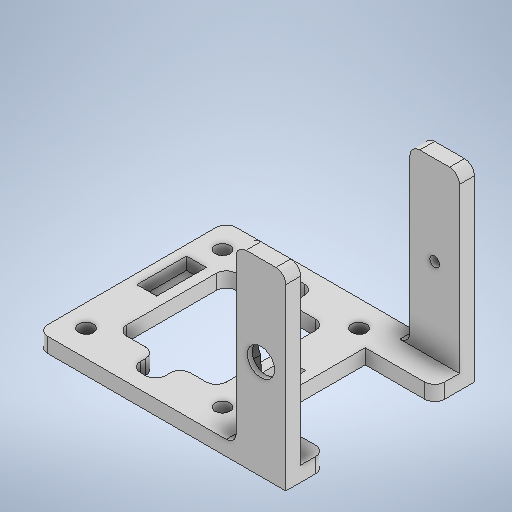
# Autodesk Inventor part: head_top
Saved by Autodesk Inventor 2026.1 (Build 301233000, 233)
## iProperties
Created: 2026-01-12
Part Number: head_top
Material: Generic
Document SubType Name: Modeling
Designer: chris
Density: 1 g/cm^3
Appearance: Default
Author: chris
Autodesk Inventor part; units mm, degrees
ref_plane "YZ Plane" through (0, 0, 0) normal (1, 0, 0) x (0, 1, 0)
ref_plane "XZ Plane" through (0, 0, 0) normal (0, 1, 0) x (-1, 0, 0)
ref_plane "XY Plane" through (0, 0, 0) normal (0, 0, 1) x (1, 0, 0)
sketch "Sketch1" plane through (0, 0, 0) normal (0, 1, 0) x (-1, 0, 0)
  line L0 (-25, 19) -> (25, 19)
  line L1 (25, 19) -> (25, -19)
  line L2 (25, -19) -> (-25, -19)
  line L3 (-25, -19) -> (-25, 19)
  line L4 (-25, 19) -> (25, -19) construction
  line L5 (25, 19) -> (-25, -19) construction
  line L6 (-15, -11) -> (25, -11)
  line L7 (25, -11) -> (25, 11)
  line L8 (25, 11) -> (-15, 11)
  line L9 (-15, 11) -> (-15, -11)
  line L10 (-15, -11) -> (25, 11) construction
  line L11 (25, -11) -> (-15, 11) construction
  point P0 (0, 0)
  point P1 (5, 0)
  point P2 (5, 0)
  point P3 (25, -11)
  point P4 (25, 11)
  dimension "d0" = 50
  dimension "d1" = 38
  dimension "d2" = 22
  dimension "d3" = 5
  dimension "d4" = 40
  constraints: 24 end point, 5 midpoint, 5 parallel, 2 perpendicular, 1 horizontal
  measures "d0" distance of L1.end L2.end
  measures "d1" distance of L0.end L1.end
  measures "d2" distance of L7.end L6.end
  measures "d3" distance of point (0, 0) point (5, 0)
  measures "d4" distance of L6.start L6.end
extrude "Extrusion1" add sketch "Sketch1" along normal blind 3 contours L0 L1 L8 L9 L6 L2 L3
sketch "Sketch2" plane through (0, 3, 0) normal (0, 1, 0) x (1, 0, 0)
  line L0 (25, -19) -> (15, -19)
  line L1 (15, -19) -> (15, -16)
  line L2 (15, -16) -> (25, -16)
  line L3 (25, -16) -> (25, -19)
  line L4 (-25, -19) -> (25, -19) projected
  line L5 (15, 11) -> (15, -11) projected
  line L6 (25, -19) -> (25, 19) projected
  line L7 (15, -11) -> (-25, -11) projected
  line L8 (15, 16) -> (25, 16)
  line L9 (25, 16) -> (25, 19)
  line L10 (25, 19) -> (15, 19)
  line L11 (15, 19) -> (15, 16)
  line L12 (-25, 11) -> (15, 11) projected
  line L13 (25, 19) -> (-25, 19) projected
  point P0 (0, 0)
  point P1 (25, 16)
  dimension "d18" = 3
  dimension "d19" = 3
  constraints: 16 end point, 6 collinear, 4 parallel, 2 horizontal, 2 perpendicular
  measures "d18" distance of L10.end L8.start
  measures "d19" distance of L0.end L1.end
extrude "Extrusion2" add sketch "Sketch2" along normal blind 35
sketch "Sketch4" plane through (25, 0, -19) normal (0, 0, -1) x (-1, 0, 0)
  circle A0 centre (5, 20) radius 1
  line L0 (0, 0) -> (50, 0) projected
  line L1 (0, 0) -> (0, 38) projected
  point P0 (25, 0)
  dimension "d20" = 2
  dimension "d21" = 20
  dimension "d22" = 5
  constraints: 1 centre point
  measures "d20" diameter of A0
  measures "d21" distance from line of A0.centre L0
  measures "d22" distance from line of L1 A0.centre
extrude "Extrusion4" cut sketch "Sketch4" against normal blind 5
sketch "Sketch6" plane through (0, 0, 0) normal (0, -1, 0) x (1, 0, 0)
  circle A0 centre (-20.5, 13.75) radius 1.5
  circle A1 centre (-20.5, -13.75) radius 1.5
  circle A2 centre (7, -13.75) radius 1.5
  circle A3 centre (7, 13.75) radius 1.5
  line L0 (-9.25, 16) -> (-4.25, 16)
  line L1 (-4.25, 16) -> (-4.25, 11)
  line L2 (-4.25, 11) -> (-9.25, 11)
  line L3 (-9.25, 11) -> (-9.25, 16)
  line L4 (-9.25, 16) -> (-4.25, 11) construction
  line L5 (-4.25, 16) -> (-9.25, 11) construction
  line L6 (15, 11) -> (-25, 11) projected
  line L7 (25, 19) -> (25, -19) projected
  line L8 (-9.25, -16) -> (-4.25, -16)
  line L9 (-4.25, -16) -> (-4.25, -11)
  line L10 (-4.25, -11) -> (-9.25, -11)
  line L11 (-9.25, -11) -> (-9.25, -16)
  line L12 (-9.25, -16) -> (-4.25, -11) construction
  line L13 (-4.25, -16) -> (-9.25, -11) construction
  line L14 (-25, -11) -> (15, -11) projected
  point P0 (0, 0)
  point P1 (-6.75, 13.5)
  point P2 (-6.75, -13.5)
  dimension "d43" = 3
  dimension "d44" = 3
  dimension "d45" = 3
  dimension "d46" = 3
  dimension "d47" = 13.75
  dimension "d48" = 13.75
  dimension "d49" = 13.75
  dimension "d50" = 13.75
  dimension "d51" = 27.5
  dimension "d52" = 27.5
  dimension "d55" = 5
  dimension "d56" = 5
  dimension "d57" = 13.75
  dimension "d58" = 18
  dimension "d59" = 18
  dimension "d60" = 5
  dimension "d61" = 5
  dimension "d62" = 13.75
  constraints: 24 end point, 4 centre point, 4 midpoint, 4 parallel, 2 collinear, 2 horizontal, 2 perpendicular
  measures "d43" diameter of A0
  measures "d44" diameter of A1
  measures "d45" diameter of A2
  measures "d46" diameter of A3
  measures "d47" vertical distance of A0.centre point (0, 0)
  measures "d48" vertical distance of point (0, 0) A1.centre
  measures "d49" vertical distance of A2.centre point (0, 0)
  measures "d50" vertical distance of A3.centre point (0, 0)
  measures "d51" distance of A2.centre A1.centre
  measures "d52" distance of A3.centre A0.centre
  measures "d55" distance of L0.end L1.end
  measures "d56" distance of L0.start L0.end
  measures "d57" horizontal distance of point (-6.75, 13.5) A0.centre
  measures "d58" distance from line of L7 A2.centre
  measures "d59" distance from line of L7 A3.centre
  measures "d60" distance of L10.end L9.end
  measures "d61" distance of L9.end L8.end
  measures "d62" horizontal distance of A2.centre point (-6.75, -13.5)
extrude "Extrusion6" cut sketch "Sketch6" against normal blind 3
sketch "Sketch7" plane through (25, 3, 16) normal (0, 0, -1) x (-1, 0, 0)
  circle A0 centre (5, 17.1114) radius 3.6
  circle A1 centre (5, 3.1114) radius 2.5
  circle A2 centre (5, 31.1114) radius 2.5
  line L0 (10, -1.5067) -> (10, 36.4933)
  line L1 (7.4901, 30.8888) -> (8.1212, 18.9054)
  line L2 (2.503, 30.9884) -> (1.9362, 19.0018)
  line L3 (2.503, 3.2345) -> (1.9362, 15.2211)
  line L4 (7.497, 3.2345) -> (8.0638, 15.2211)
  line L5 (10, 0) -> (10, 35) projected
  point P0 (25, -3)
  dimension "d63" = 7.2
  dimension "d64" = 5
  dimension "d65" = 5
  dimension "d66" = 5
  dimension "d67" = 5
  dimension "d68" = 5
  dimension "d69" = 14
  dimension "d70" = 14
  dimension "d71" = 12
  dimension "d72" = 12
  dimension "d73" = 12
  dimension "d74" = 12
  constraints: 10 end point, 8 point on circle, 3 centre point, 1 collinear
  measures "d63" diameter of A0
  measures "d64" diameter of A1
  measures "d65" diameter of A2
  measures "d66" distance from line of L0 A0.centre
  measures "d67" distance from line of L0 A1.centre
  measures "d68" distance from line of L0 A2.centre
  measures "d69" distance of A1.centre A0.centre
  measures "d70" distance of A0.centre A2.centre
  measures "d71" distance of L1.start L1.end
  measures "d72" distance of L2.start L2.end
  measures "d73" distance of L3.start L3.end
  measures "d74" distance of L4.start L4.end
extrude "Extrusion7" cut sketch "Sketch7" against normal blind 2
sketch "Sketch8" plane through (-25, 0, -11) normal (0, 0, 1) x (1, 0, 0)
  line L0 (0, 0) -> (8, 0)
  line L1 (8, 0) -> (8, 3)
  line L2 (8, 3) -> (0, 3)
  line L3 (0, 3) -> (0, 0)
  line L4 (0, 3) -> (15.75, 3) projected
  line L5 (0, 0) -> (15.75, 0) projected
  line L6 (0, 0) -> (0, 3) projected
  point P0 (25, 0)
  point P1 (8, 1.5)
  point P2 (0, 1.5)
  dimension "d77" = 8
  constraints: 8 end point, 3 collinear, 2 midpoint, 2 parallel, 1 horizontal, 1 perpendicular
  measures "d77" distance of point (8, 1.5) point (0, 1.5)
extrude "Extrusion8" add sketch "Sketch8" along normal blind 22
sketch "Sketch9" plane through (0, 0, 0) normal (0, -1, 0) x (1, 0, 0)
  line L0 (15, -11) -> (25, -11)
  line L1 (25, -11) -> (25, 11)
  line L2 (25, 11) -> (15, 11)
  line L3 (15, 11) -> (15, -11)
  line L4 (25, 19) -> (25, -19) projected
  line L5 (15, -11) -> (15, 11) projected
  line L6 (15, 11) -> (-4.25, 11) projected
  line L7 (-4.25, -11) -> (15, -11) projected
  point P0 (0, 0)
  constraints: 8 end point, 4 collinear, 2 parallel, 1 horizontal, 1 perpendicular
extrude "Extrusion9" cut sketch "Sketch9" against normal blind 3
sketch "Sketch10" plane through (25, 0, -11) normal (0, 0, 1) x (1, 0, 0)
  line L0 (-22, 0) -> (-14, 0)
  line L1 (-14, 0) -> (-14, 3)
  line L2 (-14, 3) -> (-22, 3)
  line L3 (-22, 3) -> (-22, 0)
  line L4 (-29.25, 0) -> (0, 0) projected
  line L5 (-29.25, 3) -> (0, 3) projected
  line L6 (-42, 3) -> (-42, 0) projected
  point P0 (-25, 0)
  dimension "d82" = 8
  dimension "d83" = 20
  constraints: 8 end point, 2 collinear, 2 parallel, 1 horizontal, 1 perpendicular
  measures "d82" distance between parallel lines of L1 L3
  measures "d83" distance between parallel lines of L3 L6
extrude "Extrusion10" add sketch "Sketch10" along normal blind 22
sketch "Sketch13" plane through (-25, 0, 19) normal (0, 0, 1) x (1, 0, 0)
  circle A0 centre (45, 20) radius 2.75
  line L0 (40, 38) -> (50, 38) projected
  line L1 (50, 0) -> (50, 38) projected
  point P0 (25, 0)
  dimension "d97" = 5.5
  dimension "d98" = 18
  dimension "d99" = 5
  constraints: 1 centre point
  measures "d97" diameter of A0
  measures "d98" distance from line of L0 A0.centre
  measures "d99" distance from line of L1 A0.centre
extrude "Extrusion12" cut sketch "Sketch13" against normal blind 1
sketch "Sketch14" plane through (0, 3, 0) normal (0, 1, 0) x (1, 0, 0)
  line L0 (5, -9) -> (9, -9)
  line L1 (9, -9) -> (9, 1)
  line L2 (9, 1) -> (5, 1)
  line L3 (5, 1) -> (5, -9)
  line L4 (3, 11) -> (3, -11) projected
  line L5 (3, -11) -> (-4.25, -11) projected
  point P0 (0, 0)
  dimension "d102" = 4
  dimension "d103" = 10
  dimension "d104" = 2
  dimension "d105" = 2
  constraints: 8 end point, 2 parallel, 1 horizontal, 1 perpendicular
  measures "d102" distance of L2.end L1.end
  measures "d103" distance of L1.end L0.end
  measures "d104" distance between parallel lines of L4 L3
  measures "d105" distance between parallel lines of L5 L0
extrude "Extrusion13" cut sketch "Sketch14" against normal blind 2.5
sketch "Sketch15" plane through (0, 3, 0) normal (0, 1, 0) x (1, 0, 0)
  line L0 (-23, -1) -> (-19, -1)
  line L1 (-19, -1) -> (-19, 9)
  line L2 (-19, 9) -> (-23, 9)
  line L3 (-23, 9) -> (-23, -1)
  line L4 (-25, 19) -> (-25, -19) projected
  line L5 (-17, 11) -> (-9.25, 11) projected
  point P0 (0, 0)
  dimension "d108" = 4
  dimension "d109" = 10
  dimension "d110" = 2
  dimension "d111" = 2
  constraints: 8 end point, 2 parallel, 1 horizontal, 1 perpendicular
  measures "d108" distance of L2.end L1.end
  measures "d109" distance of L1.end L0.end
  measures "d110" distance between parallel lines of L4 L3
  measures "d111" distance between parallel lines of L5 L2
extrude "Extrusion14" cut sketch "Sketch15" against normal blind 2.5
fillet "Fillet1" radius 2 22 edges at (-25, 1.5, -19) (-25, 1.5, 19) (25, 1.5, 11) (25, 1.5, -11) (25, 38, -17.5) (15, 38, -17.5) (15, 38, 17.5) (25, 38, 17.5) (3, 1.5, -11) (-4.25, 1.5, -11) (-4.25, 1.5, -16) (-9.25, 1.5, -16) (-9.25, 1.5, -11) (-17, 1.5, -11) (3, 1.5, 11) (-4.25, 1.5, 11) (-4.25, 1.5, 16) (-9.25, 1.5, 16) (-9.25, 1.5, 11) (-17, 1.5, 11) (15, 3, -17.5) (15, 3, 17.5)
body "Solid1"
